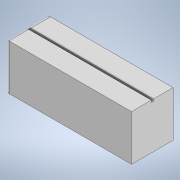
# Autodesk Inventor part: 滑盖上
Saved by Autodesk Inventor 2020 (Build 240168000, 168)
## iProperties
Created: 2021-04-06
Part Number: 滑盖上
Material: 常规
Document SubType Name: Modeling
Designer: 70929
Density: 1 g/cm^3
Appearance: 默认
Author: 70929
Autodesk Inventor part; units mm, degrees
ref_plane "YZ Plane" through (0, 0, 0) normal (1, 0, 0) x (0, 1, 0)
ref_plane "XZ Plane" through (0, 0, 0) normal (0, 1, 0) x (-1, 0, 0)
ref_plane "XY Plane" through (0, 0, 0) normal (0, 0, 1) x (1, 0, 0)
sketch "草图1" plane through (0, 0, 0) normal (0, 1, 0) x (-1, 0, 0)
  line L0 (-150, -50) -> (150, -50)
  line L1 (150, -50) -> (150, 50)
  line L2 (150, 50) -> (-150, 50)
  line L3 (-150, 50) -> (-150, -50)
  line L4 (-150, -50) -> (150, 50) construction
  line L5 (150, -50) -> (-150, 50) construction
  point P0 (0, 0)
  dimension "d0" = 300
  dimension "d1" = 100
  constraints: 12 end point, 2 midpoint, 2 parallel, 1 horizontal, 1 perpendicular
  measures "d0" distance of L2.end L1.end
  measures "d1" distance of L0.end L1.end
extrude "拉伸1" add sketch "草图1" along normal mid plane 10
sketch "草图2" plane through (0, 5, 0) normal (0, 1, 0) x (1, 0, 0)
  line L0 (-150, 50) -> (-150, -50) projected
  line L1 (150, -2.5) -> (-150, -2.5)
  line L2 (-150, -2.5) -> (-150, 2.5)
  line L3 (-150, 2.5) -> (150, 2.5)
  line L4 (150, 2.5) -> (150, -2.5)
  line L5 (150, -2.5) -> (-150, 2.5) construction
  line L6 (-150, -2.5) -> (150, 2.5) construction
  point P0 (0, 0)
  dimension "d4" = 5
  constraints: 12 end point, 2 midpoint, 2 parallel, 1 horizontal, 1 perpendicular, 1 point on line
  measures "d4" distance of L1.end L2.end
extrude "拉伸2" cut sketch "草图2" against normal blind 5
sketch "草图3" plane through (0, -5, 0) normal (0, -1, 0) x (1, 0, 0)
  line L0 (-150, 50) -> (150, 50) projected
  line L1 (150, -50) -> (-150, -50) projected
  line L2 (150, 50) -> (140, 50)
  line L3 (140, 50) -> (140, -50)
  line L4 (140, -50) -> (150, -50)
  line L5 (150, -50) -> (150, 50)
  point P0 (0, 0)
  constraints: 8 end point, 2 parallel, 1 horizontal, 1 perpendicular, 1 point on line
extrude "拉伸3" add sketch "草图3" along normal blind 100
sketch "草图4" plane through (140, -5, -50) normal (-1, 0, 0) x (0, 0, 1)
  line L0 (100, 10) -> (100, -100) projected
  line L1 (100, 0) -> (0, 0) projected
  line L2 (100, -100) -> (90, -100)
  line L3 (90, -100) -> (90, 0)
  line L4 (90, 0) -> (100, 0)
  line L5 (100, 0) -> (100, -100)
  line L6 (0, -100) -> (0, 10) projected
  line L7 (0, -100) -> (10, -100)
  line L8 (10, -100) -> (10, 0)
  line L9 (10, 0) -> (0, 0)
  line L10 (0, 0) -> (0, -100)
  point P0 (50, 5)
  constraints: 16 end point, 4 parallel, 2 horizontal, 2 perpendicular, 2 point on line
extrude "拉伸4" add sketch "草图4" along normal blind 290
fillet "圆角1" radius 5 7 edges at (-150, -55, 40) (-150, -50, 50) (-150, -55, -40) (-150, -50, -50) (-150, -5, 0) (-150, 5, -26.25) (-150, 5, 26.25)
